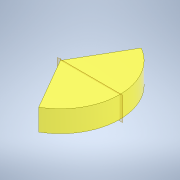
# Autodesk Inventor part: largeCap
Saved by Autodesk Inventor 2021.1 (Build 251245010, 245A)
## iProperties
Created: 2020-09-25
Part Number: largeCap
Material: PC/ABS Plastic
Document SubType Name: Modeling
Designer: robst
Density: 0.357273 g/cm^3
Appearance: Smooth - Yellow
Author: robst
Autodesk Inventor part; units mm, degrees
ref_plane "XZ Plane" through (0, 0, 0) normal (0, 1, 0) x (-1, 0, 0)
sketch "Sketch1" plane through (0, 0, 0) normal (0, 0, 1) x (1, 0, 0)
  line L0 (0, 0) -> (122.2375, 0)
  line L1 (122.2375, 0) -> (122.2375, -44.45)
  line L2 (122.2375, -44.45) -> (115.8875, -44.45)
  line L3 (115.8875, -44.45) -> (115.8875, -6.35)
  line L4 (115.8875, -6.35) -> (0, -6.35)
  line L5 (0, -6.35) -> (0, 0)
  dimension "d2" = 6.35
  dimension "d3" = 6.35
  dimension "d4" = 115.8875
  dimension "d5" = 38.1
  constraints: 12 end point, 4 perpendicular, 1 horizontal, 1 parallel
  measures "d2" distance between parallel lines of L4 L0
  measures "d3" distance between parallel lines of L1 L3
  measures "d4" distance from line of L3 L0.start
  measures "d5" distance from line of L2.end L4
revolve "Revolution1" add sketch "Sketch1" angle 120 mid plane about axis through (0, -6.35, 0) along (0, 1, 0)
ref_plane "Work Plane1" through (57.9438, -44.45, -100.3615) normal (1, 0, 0) x (0, 1, 0)
sketch "Sketch7" plane through (57.9438, -44.45, -100.3615) normal (1, 0, 0) x (0, 1, 0)
  line L0 (38.1, 0) -> (38.1, 100.3615) projected
  line L1 (44.45, 100.3615) -> (38.1, 100.3615) projected
  line L2 (44.45, 100.3615) -> (44.45, -5.4993) projected
  line L3 (44.45, -5.4993) -> (0, -5.4993) projected
  line L4 (0, -5.4993) -> (0, 0) projected
  line L5 (0, 0) -> (38.1, 0) projected
  line L6 (38.1, 0) -> (38.1, 200.723) projected
  line L7 (38.1, 100.3615) -> (38.1, 200.723) projected
  line L8 (38.1, 200.723) -> (0, 200.723) projected
  line L9 (0, 200.723) -> (0, 206.2223) projected
  line L10 (0, 206.2223) -> (44.45, 206.2223) projected
  line L11 (44.45, 206.2223) -> (44.45, 100.3615) projected
  line L12 (44.45, 100.3615) -> (38.1, 100.3615) projected
  line L13 (19.05, 0) -> (19.05, 200.723) construction
  line L14 (22.86, 143.8925) -> (22.86, 148.3076)
  line L15 (22.86, 148.3076) -> (15.24, 148.3076)
  line L16 (15.24, 148.3076) -> (15.24, 147.2949)
  line L17 (15.24, 147.2949) -> (21.9584, 147.2949)
  line L18 (21.9584, 147.2949) -> (21.9584, 143.8925)
  line L19 (21.9584, 143.8925) -> (22.86, 143.8925)
  spline S0 degree 2 poles (22.2548, 139.9837) (22.3413, 140.101) (22.65, 140.4962) (22.7427, 140.6814) knots 0 0 0 1 2 2 2
  spline S1 degree 2 poles (22.7427, 140.6814) (22.8785, 140.9346) (23.0206, 141.4101) (23.0206, 141.8424) knots 0 0 0 1 2 2 2
  spline S2 degree 2 poles (23.0206, 141.8424) (23.0206, 142.1943) (22.755, 142.8304) (22.5142, 143.0712) knots 0 0 0 1 2 2 2
  spline S3 degree 2 poles (22.5142, 143.0712) (22.2795, 143.2997) (21.5879, 143.5775) (21.2051, 143.5775) knots 0 0 0 1 2 2 2
  spline S4 degree 2 poles (21.2051, 143.5775) (20.6123, 143.5775) (19.7725, 143.0774) (19.5317, 142.534) knots 0 0 0 1 2 2 2
  spline S5 degree 2 poles (19.5317, 142.534) (19.3094, 142.0523) (19.1426, 140.7432) (19.0994, 139.9837) knots 0 0 0 1 2 2 2
  line L20 (19.0994, 139.9837) -> (18.9141, 139.9837)
  spline S6 degree 2 poles (18.9141, 139.9837) (18.5807, 139.9837) (18.167, 140.1874) (18.0496, 140.3727) knots 0 0 0 1 2 2 2
  spline S7 degree 2 poles (18.0496, 140.3727) (17.9323, 140.5579) (17.8582, 141.089) (17.8582, 141.3731) knots 0 0 0 1 2 2 2
  spline S8 degree 2 poles (17.8582, 141.3731) (17.8582, 141.7065) (18.0558, 142.6081) (18.2472, 143.0588) knots 0 0 0 1 2 2 2
  line L21 (18.2472, 143.0588) -> (18.2472, 143.1144)
  line L22 (18.2472, 143.1144) -> (17.2654, 143.1144)
  spline S9 degree 2 poles (17.2654, 143.1144) (17.1913, 142.8489) (17.0061, 141.8547) (17.0061, 141.3669) knots 0 0 0 1 2 2 2
  spline S10 degree 2 poles (17.0061, 141.3669) (17.0061, 140.7741) (17.1913, 139.9651) (17.4321, 139.644) knots 0 0 0 1 2 2 2
  spline S11 degree 2 poles (17.4321, 139.644) (17.6668, 139.3291) (18.414, 139.0204) (18.9512, 139.0204) knots 0 0 0 1 2 2 2
  line L23 (18.9512, 139.0204) -> (22.86, 139.0204)
  line L24 (22.86, 139.0204) -> (22.86, 139.9837)
  line L25 (22.86, 139.9837) -> (22.2548, 139.9837)
  line L26 (21.4521, 139.9837) -> (19.8651, 139.9837)
  spline S12 degree 2 poles (19.8651, 139.9837) (19.896, 140.3295) (20.001, 141.3731) (20.0998, 141.7003) knots 0 0 0 1 2 2 2
  spline S13 degree 2 poles (20.0998, 141.7003) (20.2171, 142.0832) (20.7049, 142.5834) (21.1372, 142.5834) knots 0 0 0 1 2 2 2
  spline S14 degree 2 poles (21.1372, 142.5834) (21.6312, 142.5834) (22.1313, 142.0276) (22.1313, 141.4966) knots 0 0 0 1 2 2 2
  spline S15 degree 2 poles (22.1313, 141.4966) (22.1313, 141.0458) (21.7423, 140.3048) (21.4521, 139.9837) knots 0 0 0 1 2 2 2
  line L27 (18.1731, 134.6361) -> (18.1731, 134.6855)
  spline S16 degree 2 poles (18.1731, 134.6855) (18.1423, 134.7966) (18.1299, 135.0375) (18.1299, 135.2042) knots 0 0 0 1 2 2 2
  spline S17 degree 2 poles (18.1299, 135.2042) (18.1299, 135.5932) (18.4695, 136.3589) (18.803, 136.7047) knots 0 0 0 1 2 2 2
  line L28 (18.803, 136.7047) -> (22.86, 136.7047)
  line L29 (22.86, 136.7047) -> (22.86, 137.668)
  line L30 (22.86, 137.668) -> (17.1419, 137.668)
  line L31 (17.1419, 137.668) -> (17.1419, 136.7047)
  line L32 (17.1419, 136.7047) -> (17.9941, 136.7047)
  spline S18 degree 2 poles (17.9941, 136.7047) (17.5248, 136.1798) (17.1419, 135.3956) (17.1419, 135.0251) knots 0 0 0 1 2 2 2
  spline S19 degree 2 poles (17.1419, 135.0251) (17.1419, 134.8769) (17.1543, 134.7287) (17.1728, 134.6361) knots 0 0 0 1 2 2 2
  line L33 (17.1728, 134.6361) -> (18.1731, 134.6361)
  spline S20 degree 2 poles (23.7739, 133.6851) (23.8171, 133.5863) (23.953, 133.2096) (24.0086, 132.9688) knots 0 0 0 1 2 2 2
  spline S21 degree 2 poles (24.0086, 132.9688) (24.0765, 132.7033) (24.1568, 132.2525) (24.1568, 131.987) knots 0 0 0 1 2 2 2
  spline S22 degree 2 poles (24.1568, 131.987) (24.1568, 131.5424) (23.9221, 130.9249) (23.7122, 130.752) knots 0 0 0 1 2 2 2
  spline S23 degree 2 poles (23.7122, 130.752) (23.5022, 130.5853) (22.9526, 130.4556) (22.6006, 130.4556) knots 0 0 0 1 2 2 2
  line L34 (22.6006, 130.4556) -> (22.1005, 130.4556)
  spline S24 degree 2 poles (22.1005, 130.4556) (22.4401, 130.8446) (22.7612, 131.5918) (22.7612, 132.1537) knots 0 0 0 1 2 2 2
  spline S25 degree 2 poles (22.7612, 132.1537) (22.7612, 133.1294) (21.3101, 134.2841) (19.9454, 134.2841) knots 0 0 0 1 2 2 2
  spline S26 degree 2 poles (19.9454, 134.2841) (19.2353, 134.2841) (18.1361, 133.8827) (17.7471, 133.5493) knots 0 0 0 1 2 2 2
  spline S27 degree 2 poles (17.7471, 133.5493) (17.3827, 133.2282) (16.9814, 132.3451) (16.9814, 131.8758) knots 0 0 0 1 2 2 2
  spline S28 degree 2 poles (16.9814, 131.8758) (16.9814, 131.4312) (17.1913, 130.7829) (17.3827, 130.4556) knots 0 0 0 1 2 2 2
  line L35 (17.3827, 130.4556) -> (17.1419, 130.4)
  line L36 (17.1419, 130.4) -> (17.1419, 129.4923)
  line L37 (17.1419, 129.4923) -> (22.2054, 129.4923)
  spline S29 degree 2 poles (22.2054, 129.4923) (23.6628, 129.4923) (25.0213, 130.7582) (25.0213, 132.0611) knots 0 0 0 1 2 2 2
  spline S30 degree 2 poles (25.0213, 132.0611) (25.0213, 132.481) (24.8854, 133.3579) (24.7743, 133.7345) knots 0 0 0 1 2 2 2
  line L38 (24.7743, 133.7345) -> (23.7739, 133.7345)
  line L39 (23.7739, 133.7345) -> (23.7739, 133.6851)
  line L40 (21.3101, 130.4556) -> (18.167, 130.4556)
  spline S31 degree 2 poles (18.167, 130.4556) (17.9941, 130.8137) (17.8459, 131.4189) (17.8459, 131.7215) knots 0 0 0 1 2 2 2
  spline S32 degree 2 poles (17.8459, 131.7215) (17.8459, 132.4501) (18.9203, 133.2899) (19.9269, 133.2899) knots 0 0 0 1 2 2 2
  spline S33 degree 2 poles (19.9269, 133.2899) (20.8778, 133.2899) (21.872, 132.6539) (21.872, 131.9376) knots 0 0 0 1 2 2 2
  spline S34 degree 2 poles (21.872, 131.9376) (21.872, 131.5609) (21.5756, 130.7705) (21.3101, 130.4556) knots 0 0 0 1 2 2 2
  spline S35 degree 2 poles (22.9897, 125.6143) (22.9897, 126.9852) (21.4521, 128.4919) (20.0318, 128.4919) knots 0 0 0 1 2 2 2
  spline S36 degree 2 poles (20.0318, 128.4919) (18.6363, 128.4919) (16.9814, 127.0284) (16.9814, 125.849) knots 0 0 0 1 2 2 2
  spline S37 degree 2 poles (16.9814, 125.849) (16.9814, 125.3179) (17.2901, 124.4967) (17.6174, 124.1941) knots 0 0 0 1 2 2 2
  spline S38 degree 2 poles (17.6174, 124.1941) (17.9447, 123.8853) (18.8894, 123.5581) (19.5749, 123.5581) knots 0 0 0 1 2 2 2
  line L41 (19.5749, 123.5581) -> (20.0998, 123.5581)
  line L42 (20.0998, 123.5581) -> (20.0998, 127.5163)
  spline S39 degree 2 poles (20.0998, 127.5163) (21.0939, 127.5163) (22.1499, 126.5159) (22.1499, 125.6267) knots 0 0 0 1 2 2 2
  spline S40 degree 2 poles (22.1499, 125.6267) (22.1499, 125.3118) (22.0078, 124.7004) (21.8967, 124.4534) knots 0 0 0 1 2 2 2
  spline S41 degree 2 poles (21.8967, 124.4534) (21.7732, 124.1941) (21.5571, 123.8359) (21.4583, 123.7186) knots 0 0 0 1 2 2 2
  line L43 (21.4583, 123.7186) -> (21.4583, 123.663)
  line L44 (21.4583, 123.663) -> (22.508, 123.663)
  spline S42 degree 2 poles (22.508, 123.663) (22.5759, 123.8298) (22.7735, 124.3361) (22.8291, 124.5337) knots 0 0 0 1 2 2 2
  spline S43 degree 2 poles (22.8291, 124.5337) (22.9094, 124.8116) (22.9897, 125.2685) (22.9897, 125.6143) knots 0 0 0 1 2 2 2
  spline S44 degree 2 poles (19.3649, 124.4967) (18.9759, 124.509) (18.4078, 124.6696) (18.2164, 124.8239) knots 0 0 0 1 2 2 2
  spline S45 degree 2 poles (18.2164, 124.8239) (18.0002, 124.9907) (17.7718, 125.5155) (17.7718, 125.9046) knots 0 0 0 1 2 2 2
  spline S46 degree 2 poles (17.7718, 125.9046) (17.7718, 126.2874) (18.0002, 126.8247) (18.2225, 127.047) knots 0 0 0 1 2 2 2
  spline S47 degree 2 poles (18.2225, 127.047) (18.451, 127.2631) (19.0006, 127.4854) (19.3649, 127.5163) knots 0 0 0 1 2 2 2
  line L45 (19.3649, 127.5163) -> (19.3649, 124.4967)
  spline S48 degree 2 poles (22.9959, 116.2592) (22.9959, 117.0002) (22.4957, 118.2537) (21.9955, 118.7107) knots 0 0 0 1 2 2 2
  spline S49 degree 2 poles (21.9955, 118.7107) (21.5015, 119.1676) (20.0195, 119.6678) (19.0562, 119.6678) knots 0 0 0 1 2 2 2
  spline S50 degree 2 poles (19.0562, 119.6678) (18.099, 119.6678) (16.6788, 119.18) (16.1539, 118.7168) knots 0 0 0 1 2 2 2
  spline S51 degree 2 poles (16.1539, 118.7168) (15.6414, 118.2599) (15.1041, 117.0125) (15.1041, 116.2406) knots 0 0 0 1 2 2 2
  spline S52 degree 2 poles (15.1041, 116.2406) (15.1041, 115.8578) (15.2153, 115.1847) (15.3018, 114.9007) knots 0 0 0 1 2 2 2
  spline S53 degree 2 poles (15.3018, 114.9007) (15.382, 114.6537) (15.6105, 114.1411) (15.7464, 113.8879) knots 0 0 0 1 2 2 2
  line L46 (15.7464, 113.8879) -> (16.969, 113.8879)
  line L47 (16.969, 113.8879) -> (16.969, 113.9682)
  spline S54 degree 2 poles (16.969, 113.9682) (16.8455, 114.1041) (16.4997, 114.524) (16.333, 114.8266) knots 0 0 0 1 2 2 2
  spline S55 degree 2 poles (16.333, 114.8266) (16.1724, 115.1168) (15.9687, 115.8022) (15.9687, 116.2468) knots 0 0 0 1 2 2 2
  spline S56 degree 2 poles (15.9687, 116.2468) (15.9687, 116.7346) (16.37, 117.6053) (16.7529, 117.9326) knots 0 0 0 1 2 2 2
  spline S57 degree 2 poles (16.7529, 117.9326) (17.1419, 118.2537) (18.3213, 118.6119) (19.0562, 118.6119) knots 0 0 0 1 2 2 2
  spline S58 degree 2 poles (19.0562, 118.6119) (19.8404, 118.6119) (20.9704, 118.2352) (21.3595, 117.9079) knots 0 0 0 1 2 2 2
  spline S59 degree 2 poles (21.3595, 117.9079) (21.7361, 117.5868) (22.119, 116.7285) (22.119, 116.2468) knots 0 0 0 1 2 2 2
  spline S60 degree 2 poles (22.119, 116.2468) (22.119, 115.8084) (21.9029, 115.0612) (21.7423, 114.771) knots 0 0 0 1 2 2 2
  spline S61 degree 2 poles (21.7423, 114.771) (21.5818, 114.4931) (21.2483, 114.0794) (21.131, 113.962) knots 0 0 0 1 2 2 2
  line L48 (21.131, 113.962) -> (21.131, 113.8879)
  line L49 (21.131, 113.8879) -> (22.3413, 113.8879)
  spline S62 degree 2 poles (22.3413, 113.8879) (22.4586, 114.1411) (22.6747, 114.5857) (22.7735, 114.9007) knots 0 0 0 1 2 2 2
  spline S63 degree 2 poles (22.7735, 114.9007) (22.8847, 115.2341) (22.9959, 115.8022) (22.9959, 116.2592) knots 0 0 0 1 2 2 2
  spline S64 degree 2 poles (22.2548, 109.8309) (22.3413, 109.9483) (22.65, 110.3435) (22.7427, 110.5287) knots 0 0 0 1 2 2 2
  spline S65 degree 2 poles (22.7427, 110.5287) (22.8785, 110.7819) (23.0206, 111.2574) (23.0206, 111.6896) knots 0 0 0 1 2 2 2
  spline S66 degree 2 poles (23.0206, 111.6896) (23.0206, 112.0416) (22.755, 112.6776) (22.5142, 112.9185) knots 0 0 0 1 2 2 2
  spline S67 degree 2 poles (22.5142, 112.9185) (22.2795, 113.1469) (21.5879, 113.4248) (21.2051, 113.4248) knots 0 0 0 1 2 2 2
  spline S68 degree 2 poles (21.2051, 113.4248) (20.6123, 113.4248) (19.7725, 112.9246) (19.5317, 112.3812) knots 0 0 0 1 2 2 2
  spline S69 degree 2 poles (19.5317, 112.3812) (19.3094, 111.8996) (19.1426, 110.5905) (19.0994, 109.8309) knots 0 0 0 1 2 2 2
  line L50 (19.0994, 109.8309) -> (18.9141, 109.8309)
  spline S70 degree 2 poles (18.9141, 109.8309) (18.5807, 109.8309) (18.167, 110.0347) (18.0496, 110.22) knots 0 0 0 1 2 2 2
  spline S71 degree 2 poles (18.0496, 110.22) (17.9323, 110.4052) (17.8582, 110.9363) (17.8582, 111.2203) knots 0 0 0 1 2 2 2
  spline S72 degree 2 poles (17.8582, 111.2203) (17.8582, 111.5538) (18.0558, 112.4553) (18.2472, 112.9061) knots 0 0 0 1 2 2 2
  line L51 (18.2472, 112.9061) -> (18.2472, 112.9617)
  line L52 (18.2472, 112.9617) -> (17.2654, 112.9617)
  spline S73 degree 2 poles (17.2654, 112.9617) (17.1913, 112.6962) (17.0061, 111.702) (17.0061, 111.2142) knots 0 0 0 1 2 2 2
  spline S74 degree 2 poles (17.0061, 111.2142) (17.0061, 110.6214) (17.1913, 109.8124) (17.4321, 109.4913) knots 0 0 0 1 2 2 2
  spline S75 degree 2 poles (17.4321, 109.4913) (17.6668, 109.1764) (18.414, 108.8676) (18.9512, 108.8676) knots 0 0 0 1 2 2 2
  line L53 (18.9512, 108.8676) -> (22.86, 108.8676)
  line L54 (22.86, 108.8676) -> (22.86, 109.8309)
  line L55 (22.86, 109.8309) -> (22.2548, 109.8309)
  line L56 (21.4521, 109.8309) -> (19.8651, 109.8309)
  spline S76 degree 2 poles (19.8651, 109.8309) (19.896, 110.1767) (20.001, 111.2203) (20.0998, 111.5476) knots 0 0 0 1 2 2 2
  spline S77 degree 2 poles (20.0998, 111.5476) (20.2171, 111.9305) (20.7049, 112.4306) (21.1372, 112.4306) knots 0 0 0 1 2 2 2
  spline S78 degree 2 poles (21.1372, 112.4306) (21.6312, 112.4306) (22.1313, 111.8749) (22.1313, 111.3438) knots 0 0 0 1 2 2 2
  spline S79 degree 2 poles (22.1313, 111.3438) (22.1313, 110.8931) (21.7423, 110.152) (21.4521, 109.8309) knots 0 0 0 1 2 2 2
  spline S80 degree 2 poles (19.8466, 102.7235) (21.2792, 102.7235) (22.9712, 104.0882) (22.9712, 105.1317) knots 0 0 0 1 2 2 2
  spline S81 degree 2 poles (22.9712, 105.1317) (22.9712, 105.5578) (22.7735, 106.2124) (22.5698, 106.552) knots 0 0 0 1 2 2 2
  line L57 (22.5698, 106.552) -> (24.9657, 106.552)
  line L58 (24.9657, 106.552) -> (24.9657, 107.5153)
  line L59 (24.9657, 107.5153) -> (17.1419, 107.5153)
  line L60 (17.1419, 107.5153) -> (17.1419, 106.552)
  line L61 (17.1419, 106.552) -> (17.7409, 106.552)
  spline S82 degree 2 poles (17.7409, 106.552) (17.4136, 106.1938) (16.9814, 105.317) (16.9814, 104.8045) knots 0 0 0 1 2 2 2
  spline S83 degree 2 poles (16.9814, 104.8045) (16.9814, 103.8226) (18.5375, 102.7235) (19.8466, 102.7235) knots 0 0 0 1 2 2 2
  spline S84 degree 2 poles (19.9577, 103.7177) (18.9759, 103.7177) (17.8953, 104.3413) (17.8953, 105.0391) knots 0 0 0 1 2 2 2
  spline S85 degree 2 poles (17.8953, 105.0391) (17.8953, 105.4467) (18.2596, 106.2124) (18.5436, 106.552) knots 0 0 0 1 2 2 2
  line L62 (18.5436, 106.552) -> (21.7917, 106.552)
  spline S86 degree 2 poles (21.7917, 106.552) (21.9708, 106.1753) (22.1066, 105.6381) (22.1066, 105.2923) knots 0 0 0 1 2 2 2
  spline S87 degree 2 poles (22.1066, 105.2923) (22.1066, 104.5451) (21.0075, 103.7177) (19.9577, 103.7177) knots 0 0 0 1 2 2 2
  spline S88 degree 2 poles (23.0082, 95.1837) (23.0082, 95.9927) (22.5142, 97.3327) (22.014, 97.8143) knots 0 0 0 1 2 2 2
  spline S89 degree 2 poles (22.014, 97.8143) (21.5077, 98.296) (20.0133, 98.8085) (19.0438, 98.8085) knots 0 0 0 1 2 2 2
  spline S90 degree 2 poles (19.0438, 98.8085) (18.1237, 98.8085) (16.6664, 98.2898) (16.1477, 97.8081) knots 0 0 0 1 2 2 2
  spline S91 degree 2 poles (16.1477, 97.8081) (15.6476, 97.345) (15.1041, 95.9865) (15.1041, 95.1776) knots 0 0 0 1 2 2 2
  spline S92 degree 2 poles (15.1041, 95.1776) (15.1041, 94.7885) (15.2153, 94.0846) (15.3141, 93.7635) knots 0 0 0 1 2 2 2
  spline S93 degree 2 poles (15.3141, 93.7635) (15.3882, 93.5041) (15.6599, 92.8743) (15.7587, 92.6829) knots 0 0 0 1 2 2 2
  line L63 (15.7587, 92.6829) -> (16.9814, 92.6829)
  line L64 (16.9814, 92.6829) -> (16.9814, 92.7693)
  spline S94 degree 2 poles (16.9814, 92.7693) (16.8146, 92.9607) (16.5121, 93.3621) (16.3392, 93.7326) knots 0 0 0 1 2 2 2
  spline S95 degree 2 poles (16.3392, 93.7326) (16.1848, 94.0414) (15.981, 94.8379) (15.981, 95.2949) knots 0 0 0 1 2 2 2
  spline S96 degree 2 poles (15.981, 95.2949) (15.981, 96.3941) (17.6359, 97.7526) (19.0129, 97.7526) knots 0 0 0 1 2 2 2
  spline S97 degree 2 poles (19.0129, 97.7526) (19.7787, 97.7526) (20.9272, 97.3944) (21.3224, 97.0548) knots 0 0 0 1 2 2 2
  spline S98 degree 2 poles (21.3224, 97.0548) (21.7176, 96.7275) (22.1313, 95.8013) (22.1313, 95.2208) knots 0 0 0 1 2 2 2
  spline S99 degree 2 poles (22.1313, 95.2208) (22.1313, 94.7947) (22.0078, 93.9426) (21.8843, 93.6523) knots 0 0 0 1 2 2 2
  line L65 (21.8843, 93.6523) -> (19.9145, 93.6523)
  line L66 (19.9145, 93.6523) -> (19.9145, 95.4184)
  line L67 (19.9145, 95.4184) -> (19.0253, 95.4184)
  line L68 (19.0253, 95.4184) -> (19.0253, 92.652)
  line L69 (19.0253, 92.652) -> (22.3536, 92.652)
  spline S100 degree 2 poles (22.3536, 92.652) (22.4401, 92.8434) (22.7056, 93.498) (22.7859, 93.7758) knots 0 0 0 1 2 2 2
  spline S101 degree 2 poles (22.7859, 93.7758) (22.8971, 94.1525) (23.0082, 94.7577) (23.0082, 95.1837) knots 0 0 0 1 2 2 2
  line L70 (22.86, 90.4722) -> (22.86, 91.4355)
  line L71 (22.86, 91.4355) -> (14.9004, 91.4355)
  line L72 (14.9004, 91.4355) -> (14.9004, 90.4722)
  line L73 (14.9004, 90.4722) -> (22.86, 90.4722)
  line L74 (22.86, 84.6121) -> (22.86, 85.5754)
  line L75 (22.86, 85.5754) -> (22.2301, 85.5754)
  spline S102 degree 2 poles (22.2301, 85.5754) (22.6192, 86.02) (23.0206, 86.8166) (23.0206, 87.3106) knots 0 0 0 1 2 2 2
  spline S103 degree 2 poles (23.0206, 87.3106) (23.0206, 87.6811) (22.7735, 88.3418) (22.508, 88.5826) knots 0 0 0 1 2 2 2
  spline S104 degree 2 poles (22.508, 88.5826) (22.2425, 88.8296) (21.4336, 89.1013) (20.8531, 89.1013) knots 0 0 0 1 2 2 2
  line L76 (20.8531, 89.1013) -> (17.1419, 89.1013)
  line L77 (17.1419, 89.1013) -> (17.1419, 88.138)
  line L78 (17.1419, 88.138) -> (20.4023, 88.138)
  spline S105 degree 2 poles (20.4023, 88.138) (20.8593, 88.138) (21.4583, 88.0701) (21.6806, 87.9528) knots 0 0 0 1 2 2 2
  spline S106 degree 2 poles (21.6806, 87.9528) (21.9029, 87.8355) (22.1066, 87.4341) (22.1066, 87.0574) knots 0 0 0 1 2 2 2
  spline S107 degree 2 poles (22.1066, 87.0574) (22.1066, 86.7054) (21.7053, 85.9088) (21.415, 85.5754) knots 0 0 0 1 2 2 2
  line L79 (21.415, 85.5754) -> (17.1419, 85.5754)
  line L80 (17.1419, 85.5754) -> (17.1419, 84.6121)
  line L81 (17.1419, 84.6121) -> (22.86, 84.6121)
  spline S108 degree 2 poles (22.9897, 80.7342) (22.9897, 82.105) (21.4521, 83.6117) (20.0318, 83.6117) knots 0 0 0 1 2 2 2
  spline S109 degree 2 poles (20.0318, 83.6117) (18.6363, 83.6117) (16.9814, 82.1482) (16.9814, 80.9688) knots 0 0 0 1 2 2 2
  spline S110 degree 2 poles (16.9814, 80.9688) (16.9814, 80.4378) (17.2901, 79.6165) (17.6174, 79.3139) knots 0 0 0 1 2 2 2
  spline S111 degree 2 poles (17.6174, 79.3139) (17.9447, 79.0051) (18.8894, 78.6779) (19.5749, 78.6779) knots 0 0 0 1 2 2 2
  line L82 (19.5749, 78.6779) -> (20.0998, 78.6779)
  line L83 (20.0998, 78.6779) -> (20.0998, 82.6361)
  spline S112 degree 2 poles (20.0998, 82.6361) (21.0939, 82.6361) (22.1499, 81.6357) (22.1499, 80.7465) knots 0 0 0 1 2 2 2
  spline S113 degree 2 poles (22.1499, 80.7465) (22.1499, 80.4316) (22.0078, 79.8202) (21.8967, 79.5732) knots 0 0 0 1 2 2 2
  spline S114 degree 2 poles (21.8967, 79.5732) (21.7732, 79.3139) (21.5571, 78.9557) (21.4583, 78.8384) knots 0 0 0 1 2 2 2
  line L84 (21.4583, 78.8384) -> (21.4583, 78.7828)
  line L85 (21.4583, 78.7828) -> (22.508, 78.7828)
  spline S115 degree 2 poles (22.508, 78.7828) (22.5759, 78.9496) (22.7735, 79.4559) (22.8291, 79.6535) knots 0 0 0 1 2 2 2
  spline S116 degree 2 poles (22.8291, 79.6535) (22.9094, 79.9314) (22.9897, 80.3884) (22.9897, 80.7342) knots 0 0 0 1 2 2 2
  spline S117 degree 2 poles (19.3649, 79.6165) (18.9759, 79.6288) (18.4078, 79.7894) (18.2164, 79.9437) knots 0 0 0 1 2 2 2
  spline S118 degree 2 poles (18.2164, 79.9437) (18.0002, 80.1105) (17.7718, 80.6354) (17.7718, 81.0244) knots 0 0 0 1 2 2 2
  spline S119 degree 2 poles (17.7718, 81.0244) (17.7718, 81.4072) (18.0002, 81.9445) (18.2225, 82.1668) knots 0 0 0 1 2 2 2
  spline S120 degree 2 poles (18.2225, 82.1668) (18.451, 82.3829) (19.0006, 82.6052) (19.3649, 82.6361) knots 0 0 0 1 2 2 2
  line L86 (19.3649, 82.6361) -> (19.3649, 79.6165)
  line L87 (22.86, 73.3056) -> (22.86, 74.2689)
  line L88 (22.86, 74.2689) -> (22.2795, 74.2689)
  spline S121 degree 2 poles (22.2795, 74.2689) (22.4648, 74.4912) (22.7118, 74.8185) (22.8168, 75.0408) knots 0 0 0 1 2 2 2
  spline S122 degree 2 poles (22.8168, 75.0408) (22.9156, 75.2445) (23.0206, 75.683) (23.0206, 75.9732) knots 0 0 0 1 2 2 2
  spline S123 degree 2 poles (23.0206, 75.9732) (23.0206, 76.4425) (22.6315, 77.2329) (22.2548, 77.5108) knots 0 0 0 1 2 2 2
  spline S124 degree 2 poles (22.2548, 77.5108) (21.8782, 77.7887) (20.7667, 78.0974) (20.0442, 78.0974) knots 0 0 0 1 2 2 2
  spline S125 degree 2 poles (20.0442, 78.0974) (19.2908, 78.0974) (18.1917, 77.7084) (17.7779, 77.3688) knots 0 0 0 1 2 2 2
  spline S126 degree 2 poles (17.7779, 77.3688) (17.4074, 77.0538) (16.9814, 76.1708) (16.9814, 75.683) knots 0 0 0 1 2 2 2
  spline S127 degree 2 poles (16.9814, 75.683) (16.9814, 75.2569) (17.1728, 74.6209) (17.3704, 74.2689) knots 0 0 0 1 2 2 2
  line L89 (17.3704, 74.2689) -> (14.9004, 74.2689)
  line L90 (14.9004, 74.2689) -> (14.9004, 73.3056)
  line L91 (14.9004, 73.3056) -> (22.86, 73.3056)
  line L92 (21.4706, 74.2689) -> (18.167, 74.2689)
  spline S128 degree 2 poles (18.167, 74.2689) (17.9941, 74.627) (17.8644, 75.1951) (17.8644, 75.5224) knots 0 0 0 1 2 2 2
  spline S129 degree 2 poles (17.8644, 75.5224) (17.8644, 76.2634) (18.9759, 77.1032) (20.0257, 77.1032) knots 0 0 0 1 2 2 2
  spline S130 degree 2 poles (20.0257, 77.1032) (21.0384, 77.1032) (22.1066, 76.461) (22.1066, 75.7509) knots 0 0 0 1 2 2 2
  spline S131 degree 2 poles (22.1066, 75.7509) (22.1066, 75.3742) (21.7608, 74.6085) (21.4706, 74.2689) knots 0 0 0 1 2 2 2
  line L93 (15.24, 63.0365) -> (22.86, 65.6609)
  line L94 (22.86, 65.6609) -> (22.86, 66.7539)
  line L95 (22.86, 66.7539) -> (15.24, 69.3783)
  line L96 (15.24, 69.3783) -> (15.24, 68.2914)
  line L97 (15.24, 68.2914) -> (21.5694, 66.1796)
  line L98 (21.5694, 66.1796) -> (15.24, 64.0677)
  line L99 (15.24, 64.0677) -> (15.24, 63.0365)
  spline S132 degree 2 poles (19.05, 57.6951) (21.1001, 57.6951) (23.0206, 58.8869) (23.0206, 60.128) knots 0 0 0 1 2 2 2
  spline S133 degree 2 poles (23.0206, 60.128) (23.0206, 61.3878) (21.0631, 62.5672) (19.0562, 62.5672) knots 0 0 0 1 2 2 2
  spline S134 degree 2 poles (19.0562, 62.5672) (16.9937, 62.5672) (15.0856, 61.3754) (15.0856, 60.128) knots 0 0 0 1 2 2 2
  spline S135 degree 2 poles (15.0856, 60.128) (15.0856, 58.8745) (17.0616, 57.6951) (19.05, 57.6951) knots 0 0 0 1 2 2 2
  spline S136 degree 2 poles (21.3718, 59.0042) (20.9951, 58.856) (19.8342, 58.7325) (19.05, 58.7325) knots 0 0 0 1 2 2 2
  spline S137 degree 2 poles (19.05, 58.7325) (18.2658, 58.7325) (17.111, 58.856) (16.722, 59.0104) knots 0 0 0 1 2 2 2
  spline S138 degree 2 poles (16.722, 59.0104) (16.333, 59.1647) (15.9316, 59.702) (15.9316, 60.128) knots 0 0 0 1 2 2 2
  spline S139 degree 2 poles (15.9316, 60.128) (15.9316, 60.5541) (16.333, 61.1037) (16.7344, 61.2643) knots 0 0 0 1 2 2 2
  spline S140 degree 2 poles (16.7344, 61.2643) (17.1234, 61.4186) (18.309, 61.5298) (19.0562, 61.5298) knots 0 0 0 1 2 2 2
  spline S141 degree 2 poles (19.0562, 61.5298) (19.8589, 61.5298) (20.9334, 61.431) (21.3533, 61.2704) knots 0 0 0 1 2 2 2
  spline S142 degree 2 poles (21.3533, 61.2704) (21.7485, 61.1222) (22.1746, 60.5726) (22.1746, 60.128) knots 0 0 0 1 2 2 2
  spline S143 degree 2 poles (22.1746, 60.128) (22.1746, 59.7081) (21.7732, 59.1586) (21.3718, 59.0042) knots 0 0 0 1 2 2 2
  line L100 (22.86, 52.0202) -> (22.86, 56.7194)
  line L101 (22.86, 56.7194) -> (21.7794, 56.7194)
  spline S144 degree 2 poles (21.7794, 56.7194) (21.3039, 56.2131) (20.4209, 55.3115) (19.9454, 54.8793) knots 0 0 0 1 2 2 2
  spline S145 degree 2 poles (19.9454, 54.8793) (18.9882, 54.0086) (17.8397, 53.3726) (17.2284, 53.3726) knots 0 0 0 1 2 2 2
  spline S146 degree 2 poles (17.2284, 53.3726) (16.9073, 53.3726) (16.4256, 53.5702) (16.2712, 53.7492) knots 0 0 0 1 2 2 2
  spline S147 degree 2 poles (16.2712, 53.7492) (16.1169, 53.9283) (15.9625, 54.3976) (15.9625, 54.6817) knots 0 0 0 1 2 2 2
  spline S148 degree 2 poles (15.9625, 54.6817) (15.9625, 54.9534) (16.0983, 55.5091) (16.2033, 55.7623) knots 0 0 0 1 2 2 2
  spline S149 degree 2 poles (16.2033, 55.7623) (16.2898, 55.9784) (16.5368, 56.3798) (16.6232, 56.5033) knots 0 0 0 1 2 2 2
  line L102 (16.6232, 56.5033) -> (16.6232, 56.5589)
  line L103 (16.6232, 56.5589) -> (15.5364, 56.5589)
  spline S150 degree 2 poles (15.5364, 56.5589) (15.382, 56.2439) (15.0794, 55.1139) (15.0794, 54.6076) knots 0 0 0 1 2 2 2
  spline S151 degree 2 poles (15.0794, 54.6076) (15.0794, 53.5393) (16.2095, 52.3351) (17.1728, 52.3351) knots 0 0 0 1 2 2 2
  spline S152 degree 2 poles (17.1728, 52.3351) (17.6236, 52.3351) (18.3769, 52.5451) (18.698, 52.7303) knots 0 0 0 1 2 2 2
  spline S153 degree 2 poles (18.698, 52.7303) (19.0315, 52.9156) (19.686, 53.4528) (20.001, 53.7492) knots 0 0 0 1 2 2 2
  spline S154 degree 2 poles (20.001, 53.7492) (20.5258, 54.2309) (21.6497, 55.4103) (21.977, 55.7623) knots 0 0 0 1 2 2 2
  line L104 (21.977, 55.7623) -> (21.977, 52.0202)
  line L105 (21.977, 52.0202) -> (22.86, 52.0202)
  constraints: 2 end point, 2 midpoint, 1 vertical
emboss "Emboss1" sketch "Sketch7" operation cut depth 1.27 direction (-1, 0, 0) wrap yes faces at (88.775, -19.05, 74.491) contours L19 L18 L17 L16 L15 L14 | L25 L24 L23 S11 S10 S9 L22 L21 S8 S7 S6 L20 S5 S4 S3 S2 S1 S0 | L33 S19 S18 L32 L31 L30 L29 L28 S17 S16 L27 | L39 L38 S30 S29 L37 L36 L35 S28 S27 S26 S25 S24 L34 S23 S22 S21 S20 | S43 S42 L44 L43 S41 S40 S39 L42 L41 S38 S37 S36 S35 | S63 S62 L49 L48 S61 S60 S59 S58 S57 S56 S55 S54 L47 L46 S53 S52 S51 S50 S49 S48 | L55 L54 L53 S75 S74 S73 L52 L51 S72 S71 S70 L50 S69 S68 S67 S66 S65 S64 | S83 S82 L61 L60 L59 L58 L57 S81 S80 | S101 S100 L69 L68 L67 L66 L65 S99 S98 S97 S96 S95 S94 L64 L63 S93 S92 S91 S90 S89 S88 | L73 L72 L71 L70 | L81 L80 L79 S107 S106 S105 L78 L77 L76 S104 S103 S102 L75 L74 | S116 S115 L85 L84 S114 S113 S112 L83 L82 S111 S110 S109 S108 | L91 L90 L89 S127 S126 S125 S124 S123 S122 S121 L88 L87 | L99 L98 L97 L96 L95 L94 L93 | S135 S134 S133 S132 | L105 L104 S154 S153 S152 S151 S150 L103 L102 S149 S148 S147 S146 S145 S144 L101 L100
sketch "Sketch8" plane through (0, 0, 0) normal (0, 0, 1) x (1, 0, 0)
  line L0 (0, 0) -> (0, -6.35) projected
  line L1 (0, -6.35) -> (57.9438, -6.35) projected
  line L2 (115.8875, -6.35) -> (57.9438, -6.35) projected
  line L3 (76.2, -3.175) -> (69.85, -3.175)
  line L4 (76.2, -3.175) -> (82.55, -3.175)
  line L5 (69.85, -3.175) -> (69.85, -6.35)
  line L6 (82.55, -3.175) -> (82.55, -6.35)
  line L7 (82.55, -6.35) -> (69.85, -6.35)
  line L8 (0, -53.34) -> (0, 8.89) projected
  point P0 (57.15, -6.35)
  dimension "d33" = 3.175
  dimension "d34" = 76.2
  dimension "d35" = 12.7
  constraints: 10 end point, 2 collinear, 2 horizontal, 2 perpendicular, 2 point on line
  measures "d33" distance between parallel lines of L3 L2
  measures "d34" horizontal distance of L3.start L0.start
  measures "d35" distance between parallel lines of L6 L5
revolve "Revolution3" cut sketch "Sketch8" angle 120 mid plane about axis through (0, 0, 0) along (0, -1, 0)
fillet "Fillet1" radius 1.5875 2 edges at (69.85, -6.35, 0) (82.55, -6.35, 0)
equation "\"d2\" = wallThickness"
equation "\"d3\" = wallThickness"
equation "\"d4\" = insideRadius"
equation "\"d5\" = height"
equation "\"d6\" = sweepAngle"
equation "\"d33\" = glueSlotHeight"
equation "\"d34\" = glueRingRadius"
equation "\"d35\" = glueSlotWidth"
equation "\"d37\" = sweepAngle"
equation "\"insideDiameter\" = 231.775"
equation "\"insideRadius\" = 0.5 * insideDiameter"
equation "\"wallThickness\" = 6.35"
equation "\"height\" = 38.1"
equation "\"sweepAngle\" = 120deg"
equation "\"glueRingDiameter\" = 152.4"
equation "\"glueRingRadius\" = 0.5 * glueRingDiameter"
equation "\"glueSlotWidth\" = 12.7"
equation "\"glueSlotHeight\" = 3.175"
body "Solid1"
